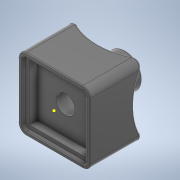
# Autodesk Inventor part: middle-centre-piece
Saved by Autodesk Inventor 2020 (Build 240168000, 168)
## iProperties
Created: 2019-10-07
Part Number: middle-centre-piece
Material: Generic
Document SubType Name: Modeling
Designer: eduso287260
Density: 1 g/cm^3
Appearance: Default
Author: eduso287260
Autodesk Inventor part; units mm, degrees
ref_plane "YZ Plane" through (0, 0, 0) normal (1, 0, 0) x (0, 1, 0)
ref_plane "XZ Plane" through (0, 0, 0) normal (0, 1, 0) x (-1, 0, 0)
sketch "Sketch3" plane through (0, 0, 0) normal (0, 0, 1) x (1, 0, 0)
  line L0 (-7.5, -9.5) -> (7.5, -9.5)
  line L1 (9.5, -7.5) -> (9.5, 7.5)
  line L2 (7.5, 9.5) -> (-7.5, 9.5)
  line L3 (-9.5, 7.5) -> (-9.5, -7.5)
  line L4 (-9.5, -9.5) -> (9.5, 9.5) construction
  line L5 (9.5, -9.5) -> (-9.5, 9.5) construction
  line L6 (-7.5, -7.5) -> (7.5, -7.5)
  line L7 (7.5, -7.5) -> (7.5, 7.5)
  line L8 (7.5, 7.5) -> (-7.5, 7.5)
  line L9 (-7.5, 7.5) -> (-7.5, -7.5)
  line L10 (-7.5, -7.5) -> (7.5, 7.5) construction
  line L11 (7.5, -7.5) -> (-7.5, 7.5) construction
  line L12 (-5.5, -5.5) -> (5.5, -5.5)
  line L13 (5.5, -5.5) -> (5.5, 5.5)
  line L14 (5.5, 5.5) -> (-5.5, 5.5)
  line L15 (-5.5, 5.5) -> (-5.5, -5.5)
  line L16 (-5.5, -5.5) -> (5.5, 5.5) construction
  line L17 (5.5, -5.5) -> (-5.5, 5.5) construction
  arc A0 (-7.5, 9.5) -> (-9.5, 7.5) centre (-7.5, 7.5) ccw
  arc A1 (-9.5, -7.5) -> (-7.5, -9.5) centre (-7.5, -7.5) ccw
  arc A2 (7.5, -9.5) -> (9.5, -7.5) centre (7.5, -7.5) ccw
  arc A3 (9.5, 7.5) -> (7.5, 9.5) centre (7.5, 7.5) ccw
  circle A4 centre (0, 0) radius 4.5
  circle A5 centre (0, 0) radius 2.5
  dimension "d8" = 19
  dimension "d9" = 19
  dimension "d10" = 15
  dimension "d11" = 15
  dimension "d12" = 11
  dimension "d13" = 11
  dimension "d20" = 2
  dimension "d21" = 9
  dimension "d22" = 5
  constraints: 36 end point, 8 point on circle, 8 point on line, 8 tangent, 6 centre point, 6 midpoint, 6 parallel, 3 equal radius, 3 horizontal, 3 perpendicular, 2 coincident
  measures "d8" distance of L5.end L4.end
  measures "d9" distance of L4.end L5.start
  measures "d10" distance of L8.end L7.end
  measures "d11" distance of L7.end L6.end
  measures "d12" distance of L14.end L13.end
  measures "d13" distance of L13.end L12.end
  measures "d20" radius of A0
  measures "d21" diameter of A4
  measures "d22" diameter of A5
ref_plane "Work Plane1" through (0, 0, 9.5) normal (0, 0, 1) x (1, 0, 0)
extrude "Extrusion7" add sketch "Sketch3" along normal blind 19 from surface at 9.5 contours A1 L3 A0 L2 A3 L1 A2 L0 | L9 L8 L7 L6 | L15 L14 L13 L12 | A4 | A5
sketch "Sketch7" plane through (0, 0, 0) normal (0, 0, 1) x (1, 0, 0)
  point P0 (0, 0)
sketch "Sketch8" plane through (-7.5, 9.5, 28.5) normal (0, 0, 1) x (1, 0, 0)
  point P0 (7.5, -9.5)
sketch "Sketch9" plane through (0, 0, 0) normal (0, 0, 1) x (1, 0, 0)
  circle A0 centre (0, 0) radius 19
  line L0 (6.3344, 17.913) -> (-6.3344, -17.913)
  dimension "d38" = 38
  constraints: 2 end point, 2 point on circle, 1 centre point, 1 coincident, 1 midpoint
  measures "d38" diameter of A0
revolve "Revolution5" cut sketch "Sketch9" angle 360 about axis through (6.3344, 17.913, 0) along (-0.3333874, -0.9427899, 0) picked at (-9.2186, 5.0677) contours L0 A0
extrude "Extrusion9" add sketch "Sketch3" along normal blind 10 from surface at 9.5 contours A4 | A5
extrude "Extrusion10" cut sketch "Sketch3" along normal blind 35.25 contours A5
fillet "Fillet2" radius 0.5 8 edges at (8.914, 8.9145, 14.2153) (0, 9.5, 16.4545) (-8.9142, 8.9143, 14.2153) (-9.5, 0, 16.4545) (-8.914, -8.9145, 14.2153) (0, -9.5, 16.4545) (8.9142, -8.9143, 14.2153) (9.5, 0, 16.4545)
fillet "Fillet3" radius 0.5 1 edges at (-4.5, 0, 9.5)
sketch "Sketch10" plane through (-7.5, 9.5, 28.5) normal (0, 0, 1) x (1, 0, 0)
  point P0 (7.5, -9.5)
sketch "Sketch12" plane through (-7.5, -9.5, 28.5) normal (0, 0, 1) x (1, 0, 0)
  line L0 (0, 2) -> (15, 2)
  line L1 (15, 2) -> (15, 17)
  line L2 (15, 17) -> (0, 17)
  line L3 (0, 17) -> (0, 2)
  line L4 (0, 2) -> (15, 17) construction
  line L5 (15, 2) -> (0, 17) construction
  line L6 (0, 1) -> (15, 1)
  line L7 (16, 2) -> (16, 17)
  line L8 (15, 18) -> (0, 18)
  line L9 (-1, 17) -> (-1, 2)
  line L10 (-1, 1) -> (16, 18) construction
  line L11 (16, 1) -> (-1, 18) construction
  arc A0 (0, 18) -> (-1, 17) centre (0, 17) ccw
  arc A1 (-1, 2) -> (0, 1) centre (0, 2) ccw
  arc A2 (15, 1) -> (16, 2) centre (15, 2) ccw
  arc A3 (16, 17) -> (15, 18) centre (15, 17) ccw
  point P0 (7.5, 9.5)
  dimension "d51" = 15
  dimension "d52" = 15
  dimension "d55" = 17
  dimension "d56" = 17
  dimension "d59" = 1
  constraints: 24 end point, 8 point on circle, 8 point on line, 8 tangent, 4 centre point, 4 midpoint, 4 parallel, 3 equal radius, 2 horizontal, 2 perpendicular
  measures "d51" distance of L2.end L1.end
  measures "d52" distance of L1.end L0.end
  measures "d55" distance of L11.end L10.end
  measures "d56" distance of L10.end L11.start
  measures "d59" radius of A0
extrude "Extrusion12" cut sketch "Sketch12" against normal blind 3 contours L3 L2 L1 L0
extrude "Extrusion13" cut sketch "Sketch12" against normal blind 1
fillet "Fillet4" radius 0.25 8 edges at (8.9142, 8.9142, 28.5) (9.5, 0, 28.5) (8.9142, -8.9142, 28.5) (0, -9.5, 28.5) (-8.9142, -8.9142, 28.5) (-9.5, 0, 28.5) (-8.9142, 8.9142, 28.5) (0, 9.5, 28.5)
fillet "Fillet5" radius 0.25 8 edges at (8.2071, 8.2071, 28.5) (8.5, 0, 28.5) (8.2071, -8.2071, 28.5) (0, -8.5, 28.5) (-8.2071, -8.2071, 28.5) (-8.5, 0, 28.5) (-8.2071, 8.2071, 28.5) (0, 8.5, 28.5)
body "Solid8"
